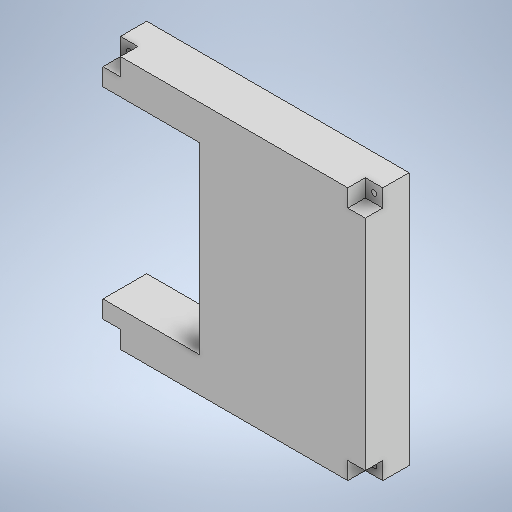
# Autodesk Inventor part: RobotBase
Saved by Autodesk Inventor 2025.3 (Build 293356000, 356)
## iProperties
Created: 2025-04-27
Part Number: RobotBase
Material: 일반
Document SubType Name: Modeling
Designer: SEON
Density: 1 g/cm^3
Appearance: 기본값
Author: SEON
Autodesk Inventor part; units mm, degrees
ref_plane "YZ Plane" through (0, 0, 0) normal (1, 0, 0) x (0, 1, 0)
ref_plane "XZ Plane" through (0, 0, 0) normal (0, 1, 0) x (-1, 0, 0)
ref_plane "XY Plane" through (0, 0, 0) normal (0, 0, 1) x (1, 0, 0)
sketch "스케치1" plane through (0, 0, 0) normal (0, 0, 1) x (1, 0, 0)
  line L0 (0, 0) -> (300, 0)
  line L1 (300, 0) -> (300, 290)
  line L2 (300, 290) -> (0, 290)
  line L3 (0, 290) -> (0, 0)
  line L4 (300, 270) -> (245, 270)
  line L5 (245, 270) -> (245, 165)
  line L6 (245, 165) -> (300, 165)
  line L7 (300, 165) -> (300, 270)
  line L8 (150, 290) -> (150, 145)
  line L9 (0, 270) -> (55, 270)
  line L10 (55, 270) -> (55, 165)
  line L11 (55, 165) -> (0, 165)
  line L12 (300, 145) -> (150, 145)
  line L13 (300, 20) -> (245, 20)
  line L14 (245, 20) -> (245, 125)
  line L15 (245, 125) -> (300, 125)
  line L16 (55, 125) -> (0, 125)
  line L17 (55, 20) -> (55, 125)
  line L18 (0, 20) -> (55, 20)
  line L19 (0, 145) -> (150, 145)
  circle A0 centre (5, 150) radius 1.5
  circle A1 centre (145, 150) radius 1.5
  circle A2 centre (5, 285) radius 1.5
  circle A3 centre (145, 285) radius 1.5
  point P0 (300, 165)
  point P1 (0, 165)
  dimension "d0" = 290
  dimension "d1" = 300
  dimension "d12" = 105
  dimension "d13" = 55
  dimension "d14" = 20
  dimension "d18" = 5
  dimension "d19" = 3
  dimension "d20" = 5
  dimension "d21" = 5
  dimension "d22" = 5
  constraints: 40 end point, 12 symmetric about line, 4 centre point, 4 horizontal, 4 parallel, 3 equal radius, 3 midpoint, 2 horizontal alignment, 2 perpendicular, 2 vertical alignment, 1 point on line, 1 vertical
  measures "d0" distance of L2.end L0.start
  measures "d1" distance of L0.start L0.end
  measures "d12" distance of L4.end L5.end
  measures "d13" distance of L5.end L6.end
  measures "d14" distance between parallel lines of L2 L4
  measures "d18" distance from line of L19 A0.centre
  measures "d19" diameter of A0
  measures "d20" distance from line of L3 A0.centre
  measures "d21" horizontal distance of L8.end A1.centre
  measures "d22" distance from line of L2 A3.centre
extrude "돌출1" add sketch "스케치1" along normal blind 25 contours L3 L11 L10 L9 L2 L8 L19
sketch "스케치3" plane through (0, 0, 25) normal (0, 0, 1) x (1, 0, 0)
  line L0 (55, 165) -> (0, 165) projected
  line L1 (0, 165) -> (0, 145) projected
  line L2 (0, 145) -> (150, 145) projected
  line L3 (150, 145) -> (150, 290) projected
  line L4 (150, 290) -> (0, 290) projected
  line L5 (0, 290) -> (0, 270) projected
  line L6 (0, 270) -> (55, 270) projected
  line L7 (55, 270) -> (55, 165) projected
  circle A0 centre (145, 285) radius 1.5 projected
  circle A1 centre (5, 285) radius 1.5 projected
  circle A2 centre (145, 150) radius 1.5 projected
  circle A3 centre (5, 150) radius 1.5 projected
  line L8 (140, 145) -> (140, 290)
  line L9 (140, 155) -> (150, 155)
  line L10 (140, 280) -> (150, 280)
  line L11 (0, 155) -> (10, 155)
  line L12 (10, 155) -> (10, 145)
  line L13 (0, 280) -> (10, 280)
  line L14 (10, 280) -> (10, 290)
  point P0 (0, 0)
  dimension "d23" = 10
  dimension "d24" = 10
  dimension "d25" = 10
  constraints: 14 end point, 8 point on line, 7 perpendicular, 2 horizontal, 2 midpoint
  measures "d23" distance between parallel lines of L4 L10
  measures "d24" distance between parallel lines of L2 L9
  measures "d25" distance between parallel lines of L3 L8
extrude "돌출3" cut sketch "스케치3" against normal blind 10 contours L11 L12 L2 L1 | L5 L4 L14 L13 | L8 L9 L3 L2 | L4 L3 L10 L8
equation "\"d20\" = d18"
equation "\"d21\" = d20"
equation "\"d22\" = d21"
